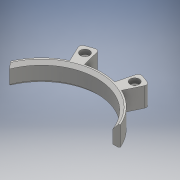
# Autodesk Inventor part: Funnel_Adapter
Saved by Autodesk Inventor 2016 (Build 200138000, 138)
## iProperties
Created: 2015-07-20
Part Number: Funnel_Adapter
Material: Generic
Document SubType Name: Modeling
Designer: bastli
Density: 1 g/cm^3
Appearance: Default
Author: bastli
Autodesk Inventor part; units mm, degrees
ref_plane "YZ Plane" through (0, 0, 0) normal (1, 0, 0) x (0, 1, 0)
ref_plane "XZ Plane" through (0, 0, 0) normal (0, 1, 0) x (-1, 0, 0)
ref_plane "XY Plane" through (0, 0, 0) normal (0, 0, 1) x (1, 0, 0)
derived "Transmission.ipt"
sketch "Sketch1" plane through (0, 0, 0) normal (0, 0, 1) x (1, 0, 0)
  circle A0 centre (-40.963, -23.65) radius 1.55 construction
  circle A1 centre (-30.4039, -36.2339) radius 1.55 construction
  circle A2 centre (-23.8046, -65.4026) radius 1.55 construction
  circle A3 centre (0, -47.3) radius 1.55 construction
  circle A4 centre (16.1776, -44.4475) radius 1.55 construction
  circle A5 centre (44.738, -53.3167) radius 1.55 construction
  circle A6 centre (40.963, -23.65) radius 1.55 construction
  circle A7 centre (-40.963, 23.65) radius 1.55 construction
  circle A8 centre (-30.4039, 36.2339) radius 1.55 construction
  circle A9 centre (-16.1776, 44.4475) radius 1.55 construction
  circle A10 centre (60.2754, 34.8) radius 1.55 construction
  circle A11 centre (44.738, 53.3167) radius 1.55 construction
  circle A12 centre (23.8046, 65.4026) radius 1.55 construction
  circle A13 centre (0, 69.6) radius 1.55 construction
  circle A14 centre (0, 47.3) radius 1.55 construction
  circle A15 centre (16.1776, 44.4475) radius 1.55 construction
  circle A16 centre (30.4039, 36.2339) radius 1.55 construction
  circle A17 centre (40.963, 23.65) radius 1.55 construction
  circle A18 centre (-23.8046, 65.4026) radius 1.55 construction
  circle A19 centre (-44.738, 53.3167) radius 1.55 construction
  circle A20 centre (-60.2754, 34.8) radius 1.55 construction
  circle A21 centre (60.2754, -34.8) radius 1.55 construction
  circle A22 centre (30.4039, -36.2339) radius 1.55 construction
  circle A23 centre (23.8046, -65.4026) radius 1.55 construction
  circle A24 centre (0, -69.6) radius 1.55 construction
  circle A25 centre (-16.1776, -44.4475) radius 1.55 construction
  circle A26 centre (-44.738, -53.3167) radius 1.55 construction
  circle A27 centre (-60.2754, -34.8) radius 1.55 construction
  circle A28 centre (69.95, 11.5) radius 2.7 construction
  circle A29 centre (46.95, -11.5) radius 2.7 construction
  circle A30 centre (-46.95, -11.5) radius 2.7 construction
  circle A31 centre (-69.95, 11.5) radius 2.7 construction
  circle A32 centre (-46.95, 11.5) radius 2.7 construction
  circle A33 centre (-69.95, -11.5) radius 2.7 construction
  circle A34 centre (46.95, 11.5) radius 2.7 construction
  circle A35 centre (69.95, -11.5) radius 2.7 construction
  circle A36 centre (-58.45, 0) radius 11.5 construction
  circle A37 centre (58.45, 0) radius 11.5 construction
  circle A38 centre (0, 0) radius 37.3 construction
  circle A39 centre (0, 0) radius 36 construction
  circle A40 centre (-58.45, 0) radius 21.46 construction
  circle A41 centre (58.45, 0) radius 21.46 construction
  circle A42 centre (-58.45, 0) radius 24.46 construction
  circle A43 centre (58.45, 0) radius 24.46 construction
  circle A44 centre (0, 0) radius 56.45 construction
  line L0 (0, 37.3) -> (0, 56.45) construction
  line L1 (0, 56.45) -> (0, 75.6) construction
  line L2 (0, 0) -> (0, 37.3) construction
  arc A45 (35.1934, 7.5778) -> (-35.1934, 7.5778) centre (0, 0) ccw
  arc A46 (50.5393, 25.1472) -> (-51.3662, 23.4118) centre (0, 0) ccw
  arc A47 (-35.1934, 7.5778) -> (-51.3662, 23.4118) centre (-58.45, 0) ccw
  arc A48 (68.7665, 31.409) -> (61.5843, 43.8491) centre (0, 0) ccw projected
  arc A49 (-68.7665, -31.409) -> (-72.8675, -20.1416) centre (-71.0408, -25.8567) ccw projected
  arc A50 (-53.8769, -53.0343) -> (-61.5843, -43.8491) centre (-57.913, -48.5947) ccw projected
  arc A51 (-53.8769, -53.0343) -> (-42.873, -62.2677) centre (0, 0) ccw projected
  arc A52 (-32.4889, -68.263) -> (-42.873, -62.2677) centre (-37.8, -65.4715) ccw projected
  arc A53 (-32.4889, -68.263) -> (-18.9906, -73.1759) centre (0, 0) ccw projected
  arc A54 (-7.1823, -75.2581) -> (-18.9906, -73.1759) centre (-13.1278, -74.4515) ccw projected
  arc A55 (-7.1823, -75.2581) -> (7.1823, -75.2581) centre (0, 0) ccw projected
  arc A56 (18.9906, -73.1759) -> (7.1823, -75.2581) centre (13.1278, -74.4515) ccw projected
  arc A57 (18.9906, -73.1759) -> (32.4889, -68.263) centre (0, 0) ccw projected
  arc A58 (42.873, -62.2677) -> (32.4889, -68.263) centre (37.8, -65.4715) ccw projected
  arc A59 (42.873, -62.2677) -> (53.8769, -53.0343) centre (0, 0) ccw projected
  arc A60 (61.5843, -43.8491) -> (53.8769, -53.0343) centre (57.913, -48.5947) ccw projected
  arc A61 (61.5843, -43.8491) -> (68.7665, -31.409) centre (0, 0) ccw projected
  arc A62 (72.8675, -20.1416) -> (68.7665, -31.409) centre (71.0408, -25.8567) ccw projected
  arc A63 (72.8675, -20.1416) -> (72.8675, 20.1416) centre (0, 0) ccw projected
  arc A64 (68.7665, 31.409) -> (72.8675, 20.1416) centre (71.0408, 25.8567) ccw projected
  arc A65 (53.8769, 53.0343) -> (61.5843, 43.8491) centre (57.913, 48.5947) ccw projected
  arc A66 (32.4889, 68.263) -> (42.873, 62.2677) centre (37.8, 65.4715) ccw projected
  arc A67 (7.1823, 75.2581) -> (18.9906, 73.1759) centre (13.1278, 74.4515) ccw projected
  arc A68 (-18.9906, 73.1759) -> (-7.1823, 75.2581) centre (-13.1278, 74.4515) ccw projected
  arc A69 (-18.9906, 73.1759) -> (-32.4889, 68.263) centre (0, 0) ccw projected
  arc A70 (-42.873, 62.2677) -> (-32.4889, 68.263) centre (-37.8, 65.4715) ccw projected
  arc A71 (-42.873, 62.2677) -> (-53.8769, 53.0343) centre (0, 0) ccw projected
  arc A72 (-61.5843, 43.8491) -> (-53.8769, 53.0343) centre (-57.913, 48.5947) ccw projected
  arc A73 (-61.5843, 43.8491) -> (-68.7665, 31.409) centre (0, 0) ccw projected
  arc A74 (-72.8675, 20.1416) -> (-68.7665, 31.409) centre (-71.0408, 25.8567) ccw projected
  arc A75 (-72.8675, 20.1416) -> (-72.8675, -20.1416) centre (0, 0) ccw projected
  arc A76 (37.3955, 12.4499) -> (-39.6914, 15.6974) centre (-1.7123, 0.6772) ccw
  line L3 (-18.2521, 38.0196) -> (-24.0357, 51.0773)
  line L4 (-10.6813, 40.5216) -> (-13.8768, 54.7178)
  arc A77 (50.982, 23.2921) -> (35.1934, 7.5778) centre (58.45, 0) ccw
  line L5 (10.0716, 39.7816) -> (14.5221, 54.5501)
  line L6 (24.5983, 50.8087) -> (17.2673, 36.8406)
  arc A78 (53.8769, 53.0343) -> (42.873, 62.2677) centre (0, 0) ccw projected
  arc A79 (-68.7665, -31.409) -> (-61.5843, -43.8491) centre (0, 0) ccw projected
  arc A80 (32.4889, 68.263) -> (18.9906, 73.1759) centre (0, 0) ccw projected
  arc A81 (7.1823, 75.2581) -> (-7.1823, 75.2581) centre (0, 0) ccw projected
  point P0 (0, 47.3)
  point P1 (-30.4039, 36.2339)
  point P2 (30.4039, 36.2339)
  point P3 (30.4039, -36.2339)
  point P4 (0, -47.3)
  point P5 (-30.4039, -36.2339)
  point P6 (0, 0)
  point P7 (0, 0)
  dimension "d0" = 72
  dimension "d3" = 42.92
  dimension "d4" = 42.92
  dimension "d6" = 3
  dimension "d7" = 3
  dimension "d33" = 3
  dimension "d34" = 4.5
  dimension "d35" = 4.5
  dimension "d36" = 4.5
  dimension "d37" = 4.5
  constraints: 29 point on circle, 20 coincident, 14 end point, 9 centre point, 4 line through centre, 2 vertical, 1 collinear, 1 point on line, 1 vertical alignment, 7 other
  measures "d3" diameter of A40
  measures "d4" diameter of A41
  measures "d6" radial gap between concentric circles of A40 A42
  measures "d34" distance from line of L4 A9.centre
  measures "d35" distance from line of L3 A9.centre
  measures "d36" distance from line of A15.centre L5
  measures "d37" distance from line of L6 A15.centre
extrude "Extrusion1" add sketch "Sketch1" along normal blind 12.7 contours A45 A47 A76 A77 | A76 L5 A46 L6 | L3 A46 L4 A76
sketch "Sketch2" plane through (0, 0, 12.7) normal (0, 0, 1) x (1, 0, 0)
  circle A0 centre (-30.4039, 36.2339) radius 1.55 projected
  circle A1 centre (-16.1776, 44.4475) radius 1.55 projected
  circle A2 centre (0, 47.3) radius 1.55 projected
  circle A3 centre (16.1776, 44.4475) radius 1.55 projected
  circle A4 centre (30.4039, 36.2339) radius 1.55 projected
  point P0 (0, 0)
  constraints: 5 coincident
hole "Hole1" at (-30.4039, 36.2339, 12.7) at (0, 47.3, 12.7) at (30.4039, 36.2339, 12.7) at (16.1776, 44.4475, 12.7) at (-16.1776, 44.4475, 12.7) direction (0, 0, -1) diameter 3.1 end through all
hole "Hole2" at (-30.4039, 36.2339, 12.7) at (-16.1776, 44.4475, 12.7) at (0, 47.3, 12.7) at (16.1776, 44.4475, 12.7) at (30.4039, 36.2339, 12.7) direction (0, 0, -1) diameter 6 depth 3
chamfer "Chamfer1" distance 2 angle 45 1 edges at (0, 36, 0)
chamfer "Chamfer2" distance 2 angle 45 1 edges at (0, 36, 12.7)
fillet "Fillet1" radius 2 4 edges at (24.5983, 50.8087, 6.35) (14.5221, 54.5501, 6.35) (-13.8768, 54.7178, 6.35) (-24.0357, 51.0773, 6.35)
equation "\"d0\" = funnel_width"
equation "\"d3\" = d5"
equation "\"d4\" = d5"
equation "\"d7\" = thickness"
equation "\"d33\" = thickness"
equation "\"d34\" = 1.5 * thickness"
equation "\"d35\" = 1.5 * thickness"
equation "\"d36\" = 1.5 * thickness"
equation "\"d37\" = 1.5 * thickness"
equation "\"funnel_width\" = 72"
equation "\"thickness\" = 3"
equation "\"d5\" = 42.92"
body "Solid1"
